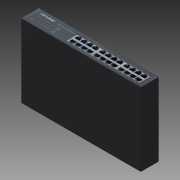
# Autodesk Inventor part: tl_sg1024
Saved by Autodesk Inventor 2013 SP2 (Build 170200200, 200)
## iProperties
Created: 2018-09-04
Part Number: tl_sg1024
Material: Generic
Document SubType Name: Modeling
Designer: alex
Density: 1 g/cm^3
Mass: 2328.35 g
Surface Area: 1477.25 cm^2
Volume: 2328.35 cm^3
GlobalPropertyList: <PropertyList/>
Author: alex
Autodesk Inventor part; units mm, degrees
ref_plane "YZ Plane" through (0, 0, 0) normal (1, 0, 0) x (0, 1, 0)
ref_plane "XZ Plane" through (0, 0, 0) normal (0, 1, 0) x (-1, 0, 0)
ref_plane "XY Plane" through (0, 0, 0) normal (0, 0, 1) x (1, 0, 0)
sketch "Sketch1" plane through (0, 0, 0) normal (0, 1, 0) x (-1, 0, 0)
  line L0 (-147, -90) -> (147, -90)
  line L1 (147, -90) -> (147, 90)
  line L2 (147, 90) -> (-147, 90)
  line L3 (-147, 90) -> (-147, -90)
  line L4 (-147, -90) -> (147, 90) construction
  line L5 (147, -90) -> (-147, 90) construction
  point P0 (0, 0)
  dimension "d0" = 294
  dimension "d1" = 180
  constraints: 12 end point, 2 midpoint, 2 parallel, 1 horizontal, 1 perpendicular
  measures "d0" distance of L2.end L1.end
  measures "d1" distance of L1.end L0.end
extrude "Extrusion1" add sketch "Sketch1" along normal blind 44
sketch "Sketch3" plane through (0, 0, 0) normal (0, -1, 0) x (1, 0, 0)
  line L0 (147, -90) -> (-147, -90) projected
  line L1 (147, 90) -> (147, -90) projected
  line L2 (-147, 90) -> (147, 90) projected
  line L3 (-147, -90) -> (-147, 90) projected
  point P0 (0, 0)
  point P1 (-140, 60.5)
  point P2 (30, -78)
  point P3 (138.5, 63)
  dimension "d7" = 7
  dimension "d8" = 29.5
  dimension "d9" = 12
  dimension "d11" = 117
  dimension "d12" = 8.5
  dimension "d13" = 27
  measures "d7" distance from line of L3 point (-140, 60.5)
  measures "d8" distance from line of L2 point (-140, 60.5)
  measures "d9" distance from line of L0 point (30, -78)
  measures "d11" distance from line of L1 point (30, -78)
  measures "d12" distance from line of L1 point (138.5, 63)
  measures "d13" distance from line of L2 point (138.5, 63)
hole "Hole1" at (-140, 0, 60.5) at (30, 0, -78) at (138.5, 0, 63) direction (0, 1, 0) diameter 3 depth 6 tip angle 118
body "Solid1"
